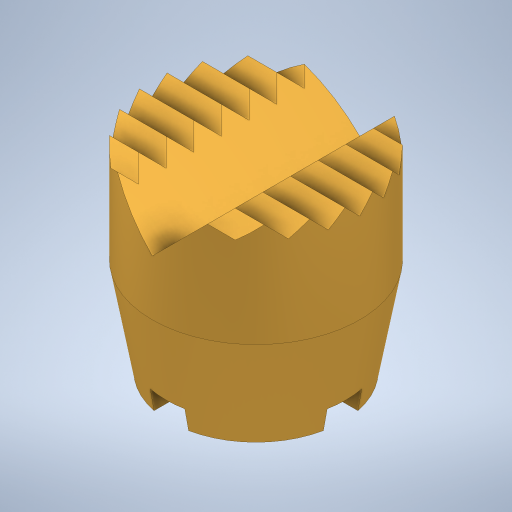
# Autodesk Inventor part: CHAPEU
Saved by Autodesk Inventor 2024 (Build 280153000, 153)
## iProperties
Created: 2023-05-08
Part Number: CHAPEU
Material: Latão, amarelo macio
Document SubType Name: Modeling
Designer: ANDRÉ
Mass: 111.06 g
Surface Area: 47.0859 cm^2
Volume: 13.1122 cm^3
Density: 8.47 g/cm^3
Appearance: Latão - Acetinado
Author: ANDRÉ
Autodesk Inventor part; units mm, degrees
ref_plane "YZ Plane" through (0, 0, 0) normal (1, 0, 0) x (0, 1, 0)
ref_plane "XZ Plane" through (0, 0, 0) normal (0, 1, 0) x (-1, 0, 0)
ref_plane "XY Plane" through (0, 0, 0) normal (0, 0, 1) x (1, 0, 0)
sketch "Esboço1" plane through (0, 0, 0) normal (1, 0, 0) x (0, 1, 0)
  line L0 (0, 0) -> (29, 0)
  line L1 (29, 0) -> (29, -15)
  line L2 (29, -15) -> (14, -15)
  line L3 (14, -15) -> (0, -12.5)
  line L4 (0, -12.5) -> (0, -9)
  line L5 (0, -9) -> (9.7213, -9)
  arc A0 (9, -9) -> (18, 0) centre (9, 0) ccw
  point P0 (4.8606, -9)
  dimension "d0" = 15
  dimension "d1" = 12.5
  dimension "d2" = 15
  dimension "d3" = 29
  dimension "d5" = 9
  dimension "d7" = 9
  constraints: 12 end point, 3 perpendicular, 3 point on line, 2 point on circle, 1 centre point, 1 horizontal, 1 midpoint, 1 parallel
  measures "d0" distance between parallel lines of L0 L2
  measures "d1" distance from line of L3.end L0
  measures "d2" distance of L1.end L2.end
  measures "d3" distance of L0.start L0.end
  measures "d5" distance from line of point (4.861, -9) L0
  measures "d7" distance from line of L4 A0.centre
revolve "Revolução1" add sketch "Esboço1" angle 360 about axis through (0, 0, 0) along (0, 1, 0)
sketch "Esboço2" plane through (0, 0, 0) normal (0, 0, 1) x (1, 0, 0)
  line L0 (0, 0) -> (0, 39.2335)
  line L1 (-2.5, 3) -> (2.5, 3)
  line L2 (2.5, 3) -> (2.5, -0.6056)
  line L3 (2.5, -0.6056) -> (-2.5, -0.6056)
  line L4 (-2.5, -0.6056) -> (-2.5, 3)
  line L5 (12.5, 0) -> (-12.5, 0) projected
  dimension "d9" = 5
  dimension "d10" = 2.5
  dimension "d11" = 3
  constraints: 10 end point, 2 parallel, 1 horizontal, 1 perpendicular, 1 vertical
  measures "d9" distance of L2.end L3.end
  measures "d10" distance between parallel lines of L2 L0
  measures "d11" distance between parallel lines of L5 L1
extrude "Extrusão1" cut sketch "Esboço2" along normal through all both and the other way through all
pattern_circular "Padrão circular1" count 4 over 360 about axis through (0, 21.5, 0) along (0, 1, 0) of "Extrusão1"
sketch "Esboço3" plane through (0, 0, 0) normal (0, 0, 1) x (1, 0, 0)
  line L0 (15, 29) -> (-15, 29) projected
  line L1 (-7, 29) -> (0, 22)
  line L2 (0, 22) -> (7, 29)
  line L3 (-7, 29) -> (7, 29)
  line L4 (0, 29) -> (0, 9.5937)
  line L5 (2.5, 0) -> (2.5, 3) projected
  point P0 (0, 0)
  dimension "d17" = 45
  dimension "d19" = 2.5
  dimension "d20" = 7
  constraints: 8 end point, 3 point on line, 2 perpendicular, 1 collinear, 1 midpoint
  measures "d17" angle of L4 L2
  measures "d19" distance between parallel lines of L5 L4
  measures "d20" distance from line of L0 L1.end
extrude "Extrusão2" cut sketch "Esboço3" along normal through all both and the other way through all
sketch "Esboço4" plane through (0, 0, 0) normal (1, 0, 0) x (0, 1, 0)
  line L0 (29, -13.2665) -> (29, 13.2665) projected
  line L1 (29, -2) -> (27, 0)
  line L2 (27, 0) -> (29, 2)
  line L3 (29, -2) -> (29, 2)
  line L4 (3, -2.5) -> (3, 2.5) projected
  line L5 (3, 0) -> (30.8136, 0)
  point P0 (0, 0)
  dimension "d23" = 2
  dimension "d24" = 45
  dimension "d25" = 45
  constraints: 8 end point, 3 point on line, 1 collinear, 1 horizontal, 1 midpoint
  measures "d23" distance from line of L1.end L0
  measures "d24" angle of L5 L1
  measures "d25" angle of L5 L2
extrude "Extrusão3" cut sketch "Esboço4" along normal through all both and the other way through all
pattern_linear "Padrão retangular1" count 4 spacing 4 along (0, 0, 1) of "Extrusão3"
pattern_linear "Padrão retangular2" count 4 spacing 4 along (0, 0, -1) of "Extrusão3"
